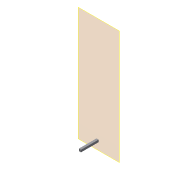
# Autodesk Inventor part: supports
Saved by Autodesk Inventor 2020 (Build 240168000, 168)
## iProperties
Created: 2019-11-23
Part Number: supports
Material: Generic
Document SubType Name: Modeling
Designer: ball
Density: 1 g/cm^3
Appearance: Default
Author: ball
Autodesk Inventor part; units mm, degrees
ref_plane "YZ Plane" through (0, 0, 0) normal (1, 0, 0) x (0, 1, 0)
ref_plane "XZ Plane" through (0, 0, 0) normal (0, 1, 0) x (-1, 0, 0)
ref_plane "XY Plane" through (0, 0, 0) normal (0, 0, 1) x (1, 0, 0)
ref_plane "Work Plane1" through (0, 0, 0) normal (0, 0, 1) x (1, 0, 0)
sketch "Sketch1" plane through (0, 0, 0) normal (0, 0, 1) x (1, 0, 0)
  circle A0 centre (-5.3931, -215.9272) radius 1.778 construction
  line L0 (-0.6306, -211.1647) -> (-10.1556, -211.1647)
  line L1 (-10.1556, -211.1647) -> (-10.1556, -220.6897)
  line L2 (-10.1556, -220.6897) -> (-0.6306, -220.6897)
  line L3 (-0.6306, -220.6897) -> (-0.6306, -211.1647)
  line L4 (-0.6306, -211.1647) -> (-10.1556, -220.6897) construction
  line L5 (-10.1556, -211.1647) -> (-0.6306, -220.6897) construction
  circle A1 centre (-5.3931, -215.9272) radius 1.5494
  point P0 (0, 0)
  dimension "d0" = 9.525
  dimension "d1" = 9.525
  dimension "d2" = 3.0988
  constraints: 12 end point, 2 midpoint, 2 parallel, 1 centre point, 1 coincident, 1 horizontal, 1 perpendicular
  measures "d0" distance of L2.end L1.end
  measures "d1" distance of L1.end L0.end
  measures "d2" diameter of A1
ref_plane "Work Plane2" through (-150.1545, -254.8124, 77.677) normal (0, 0, -1) x (0, 1, 0)
extrude "Extrusion1" add sketch "Sketch1" along normal up to surface (77.677 mm away)
body "Solid1"
